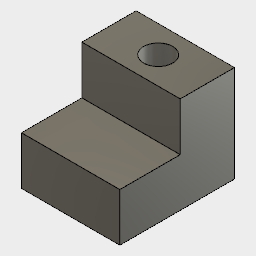
Pelvis Stump (Autodesk Fusion 360 design; units mm, degrees)
Autodesk Fusion 360 part; units mm, degrees
sketch "Sketch1" plane through (0, 0, 0) normal (0, 1, 0) x (1, 0, 0)
  line L0 (0, 0) -> (8.15, 0)
  line L1 (8.15, 0) -> (8.15, -4.5)
  line L2 (0, 0) -> (0, -4.5)
  line L3 (8.15, -4.5) -> (0, -4.5)
  line L4 (4.075, 0) -> (4.075, -4.5)
  circle A0 centre (4.075, -2.25) radius 1.75
  dimension "d1" = 8.15
  dimension "d2" = 4.5
  dimension "d3" = 4.5
  dimension "d4" = 3.5
  measures "d1" distance of L0.start L0.end
  measures "d2" distance of L0.end L1.end
  measures "d3" distance of L0.start L2.end
  measures "d4" diameter of A0
extrude "Extrude1" add sketch "Sketch1" along normal blind 8 contours L0 L2 L3 L4 A0 | L0 L1 L3 L4 A0
sketch "Sketch2" plane through (0, 0, 4.5) normal (0, 0, 1) x (1, 0, 0)
  line L0 (0, 0) -> (8.15, 0)
  line L1 (8.15, 0) -> (8.15, 8)
  line L2 (8.15, 8) -> (0, 8)
  line L3 (0, 8) -> (0, 0)
  line L4 (0, 8) -> (0, 3.5)
  line L5 (0, 3.5) -> (0, 0)
  line L6 (0, 4) -> (8.15, 4)
  line L7 (8.15, 4) -> (8.15, 0)
  line L8 (8.15, 0) -> (0, 0)
  dimension "d7" = 4.5
  measures "d7" distance of L2.end L4.end
extrude "Extrude2" add sketch "Sketch2" along normal blind 5 contours L0 L1 L3 L4 L5 L6 L7 L8
sketch "Sketch3" plane through (0, 8, 0) normal (0, 1, 0) x (-1, 0, 0)
  circle A0 centre (-4.075, 2.25) radius 1.75
  line L0 (0, 0) -> (0, 4.5)
  line L1 (0, 4.5) -> (-8.15, 4.5)
  line L2 (-8.15, 4.5) -> (-8.15, 0)
  line L3 (-8.15, 0) -> (0, 0)
  circle A1 centre (-4.075, 2.25) radius 1
  dimension "d10" = 2
  measures "d10" diameter of A1
extrude "Extrude3" add sketch "Sketch3" against normal blind 8 contours A0
sketch "Sketch4" plane through (0, 8, 0) normal (0, 1, 0) x (-1, 0, 0)
  circle A0 centre (-4.075, 2.25) radius 1
  line L0 (0, 0) -> (0, 4.5)
  line L1 (0, 4.5) -> (-8.15, 4.5)
  line L2 (-8.15, 4.5) -> (-8.15, 0)
  line L3 (-8.15, 0) -> (0, 0)
  circle A1 centre (-4.075, 2.25) radius 0.75
  dimension "d13" = 1.5
  measures "d13" diameter of A1
extrude "Extrude4" add sketch "Sketch4" against normal blind 8 contours A0
sketch "Sketch5" plane through (0, 8, 0) normal (0, 1, 0) x (-1, 0, 0)
  circle A0 centre (-4.075, 2.25) radius 0.75
  line L0 (0, 0) -> (0, 4.5)
  line L1 (0, 4.5) -> (-8.15, 4.5)
  line L2 (-8.15, 4.5) -> (-8.15, 0)
  line L3 (-8.15, 0) -> (0, 0)
  circle A1 centre (-4.075, 2.25) radius 1.2
  dimension "d17" = 2.4
  measures "d17" diameter of A1
extrude "Extrude5" cut sketch "Sketch5" against normal blind 20 contours A1
equation "HoleDiameter = 2 mm"
